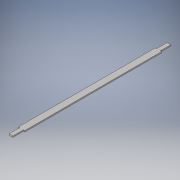
# Autodesk Inventor part: front
Saved by Autodesk Inventor 2016 SP2 (Build 200236200, 236)
## iProperties
Created: 2017-09-04
Part Number: front
Material: Generic
Document SubType Name: Modeling
Designer: Kartikye
Density: 1 g/cm^3
Appearance: Default
Author: Kartikye
Autodesk Inventor part; units mm, degrees
ref_plane "YZ Plane" through (0, 0, 0) normal (1, 0, 0) x (0, 1, 0)
ref_plane "XZ Plane" through (0, 0, 0) normal (0, 1, 0) x (-1, 0, 0)
ref_plane "XY Plane" through (0, 0, 0) normal (0, 0, 1) x (1, 0, 0)
sketch "Sketch1" plane through (0, 0, 0) normal (0, 1, 0) x (-1, 0, 0)
  line L0 (3.175, 0) -> (3.175, 165.1)
  line L1 (3.175, 165.1) -> (0, 165.1)
  line L2 (0, 165.1) -> (0, 190.5)
  line L3 (0, 190.5) -> (-8.89, 190.5)
  line L4 (-8.89, 190.5) -> (-8.89, 165.1)
  line L5 (-8.89, 165.1) -> (-12.065, 165.1)
  line L6 (-12.065, 165.1) -> (-12.065, -165.1)
  line L7 (-12.065, -165.1) -> (-8.89, -165.1)
  line L8 (-8.89, -165.1) -> (-8.89, -190.5)
  line L9 (-8.89, -190.5) -> (0, -190.5)
  line L10 (0, -190.5) -> (0, -165.1)
  line L11 (0, -165.1) -> (3.175, -165.1)
  line L12 (3.175, -165.1) -> (3.175, 0)
  point P0 (0, 0)
  dimension "d0" = 165.1
  dimension "d1" = 3.175
  dimension "d2" = 25.4
  dimension "d3" = 8.89
  dimension "d4" = 25.4
  dimension "d5" = 3.175
  dimension "d6" = 90
  dimension "d7" = 330.2
  dimension "d8" = 3.175
  dimension "d9" = 25.4
  dimension "d10" = 8.89
  dimension "d11" = 25.4
  dimension "d12" = 3.175
  constraints: 26 end point, 6 perpendicular, 6 point on line, 1 vertical
  measures "d0" distance of L0.start L0.end
  measures "d1" distance of L0.end L1.end
  measures "d2" distance of L1.end L2.end
  measures "d3" distance of L2.end L3.end
  measures "d4" distance of L3.end L4.end
  measures "d5" distance of L4.end L5.end
  measures "d6" angle of L4 L5
  measures "d7" distance of L5.end L6.end
  measures "d8" distance of L6.end L7.end
  measures "d9" distance of L7.end L8.end
  measures "d10" distance of L8.end L9.end
  measures "d11" distance of L9.end L10.end
  measures "d12" distance of L10.end L11.end
extrude "Extrusion1" add sketch "Sketch1" along normal blind 3.175
body "Solid1"
